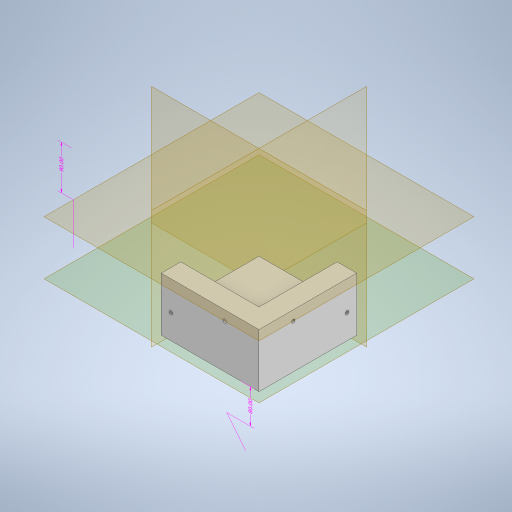
# Autodesk Inventor part: container_back_head_2
Saved by Autodesk Inventor 2023 (Build 270158000, 158)
## iProperties
Created: 2022-10-30
Part Number: container_back_head_2
Material: Genérico
Document SubType Name: Modeling
Designer: papel
Density: 1 g/cm^3
Appearance: Valor por defecto
Surface Area: 1564.19 cm^2
Author: papel
Autodesk Inventor part; units mm, degrees
ref_plane "YZ Plane" through (0, 0, 0) normal (1, 0, 0) x (0, 1, 0)
ref_plane "XZ Plane" through (0, 0, 0) normal (0, 1, 0) x (-1, 0, 0)
ref_plane "XY Plane" through (0, 0, 0) normal (0, 0, 1) x (1, 0, 0)
sketch "Boceto2" plane through (0, 0, 0) normal (0, 1, 0) x (-1, 0, 0)
  line L0 (7.5, 100) -> (-7.5, 100)
  line L1 (-7.5, 100) -> (-7.5, -100)
  line L2 (-7.5, -100) -> (7.5, -100)
  line L3 (7.5, -100) -> (7.5, 100)
  line L4 (7.5, 100) -> (-7.5, -100) construction
  line L5 (-7.5, 100) -> (7.5, -100) construction
  point P0 (0, 0)
  dimension "d7" = 15
  dimension "d8" = 200
  constraints: 12 end point, 2 midpoint, 2 parallel, 1 horizontal, 1 perpendicular
  measures "d7" distance of L2.end L1.end
  measures "d8" distance of L1.end L0.end
extrude "Extrusión1" add sketch "Boceto2" along normal blind 10
sketch "Boceto3" plane through (0, 10, 0) normal (0, 1, 0) x (1, 0, 0)
  line L0 (5, 60) -> (-5, 60)
  line L1 (-5, 60) -> (-5, 70)
  line L2 (-5, 70) -> (5, 70)
  line L3 (5, 70) -> (5, 60)
  line L4 (5, 60) -> (-5, 70) construction
  line L5 (7.5, 100) -> (-7.5, 100) projected
  line L6 (0, 64.5148) -> (0, 61.9205)
  circle A0 centre (3.25, 61.75) radius 1.75
  circle A1 centre (-3.25, 68.25) radius 1.75
  line L7 (-7.5, 100) -> (-7.5, -100) projected
  line L8 (-7.5, 0) -> (0, 0)
  line L9 (5, -70) -> (5, -60)
  line L10 (-5, -70) -> (5, -70)
  line L11 (5, -60) -> (-5, -60)
  line L12 (-5, -60) -> (-5, -70)
  line L13 (5, -60) -> (-5, -70) construction
  line L14 (0, -64.5148) -> (0, -61.9205)
  circle A2 centre (-3.25, -68.25) radius 1.75
  circle A3 centre (3.25, -61.75) radius 1.75
  point P0 (3.25, 68.25)
  point P1 (-5, 65)
  point P2 (-3.25, 61.75)
  point P3 (0, 100)
  point P4 (3.25, -68.25)
  point P5 (-3.25, -61.75)
  point P6 (-5, -65)
  dimension "d12" = 1.75
  dimension "d13" = 1.75
  dimension "d14" = 1.75
  dimension "d15" = 1.75
  dimension "d16" = 10
  dimension "d17" = 10
  dimension "d19" = 30
  dimension "d67" = 31.75
  constraints: 26 end point, 13 symmetric about line, 4 centre point, 3 midpoint, 2 horizontal, 2 parallel, 1 perpendicular, 1 vertical, 2 other
  measures "d12" distance from line of L2 point (3.25, 68.25)
  measures "d13" distance from line of L3 point (3.25, 68.25)
  measures "d14" distance from line of L1 point (-3.25, 61.75)
  measures "d15" distance from line of L0 point (-3.25, 61.75)
  measures "d16" distance between parallel lines of L0 L2
  measures "d17" distance between parallel lines of L3 L1
  measures "d19" distance from line of point (0, 100) L2
  measures "d67" distance from line of L5 A1.centre
hole "Agujero1" at (3.25, 10, -61.75) at (-3.25, 10, -68.25) at (-3.25, 10, 68.25) at (3.25, 10, 61.75) direction (0, -1, 0) diameter 3.5 end through all
sketch "Boceto4" plane through (0, 10, 0) normal (0, 1, 0) x (1, 0, 0)
  line L0 (-7.5, 100) -> (-7.5, -100) projected
  line L1 (-7.5, -100) -> (7.5, -100)
  line L2 (7.5, -100) -> (7.5, -80)
  line L3 (7.5, -80) -> (-7.5, -80)
  line L4 (-7.5, -80) -> (-7.5, -100)
  line L5 (-7.5, 0) -> (1.0116, 0)
  line L6 (-7.5, -100) -> (-7.5, 100)
  line L7 (-7.5, 100) -> (7.5, 100)
  line L8 (7.5, 100) -> (7.5, 80)
  line L9 (7.5, 80) -> (-7.5, 80)
  line L10 (-7.5, 80) -> (-7.5, 100)
  point P0 (0, 0)
  point P1 (-7.5, -80)
  point P2 (-7.5, 80)
  dimension "d27" = 15
  dimension "d28" = 20
  constraints: 20 end point, 5 symmetric about line, 2 horizontal, 2 parallel, 1 midpoint, 1 perpendicular
  measures "d27" distance of L3.end L2.end
  measures "d28" distance of L2.end L1.end
extrude "Extrusión2" add sketch "Boceto4" along normal blind 80
sketch "Boceto5" plane through (0, 90, 0) normal (0, 1, 0) x (1, 0, 0)
  line L0 (-7.5, -100) -> (7.5, -100) projected
  line L1 (-7.5, -100) -> (40.5, -100)
  line L2 (40.5, -100) -> (40.5, 100)
  line L3 (40.5, 100) -> (-7.5, 100)
  line L4 (-7.5, 100) -> (-7.5, -100)
  line L5 (40.5, -100) -> (-159.5, -100)
  line L6 (-159.5, -100) -> (-159.5, 100)
  line L7 (-159.5, 100) -> (40.5, 100)
  line L8 (40.5, 100) -> (40.5, -100)
  point P0 (0, 0)
  point P1 (-7.5, 100)
  dimension "d31" = 48
  dimension "d32" = 200
  dimension "d74" = 200
  constraints: 16 end point, 4 parallel, 2 horizontal, 2 perpendicular, 1 point on line
  measures "d31" distance of L3.end L2.end
  measures "d32" distance of L6.end L7.end
  measures "d74" distance between parallel lines of L7 L5
extrude "Extrusión3" add sketch "Boceto5" along normal blind 110
sketch "Boceto6" plane through (0, 200, 0) normal (0, 1, 0) x (1, 0, 0)
  line L0 (40.5, 100) -> (7.5, 100) projected
  line L1 (40.5, 100) -> (20.5, 100)
  line L2 (20.5, 100) -> (20.5, 80)
  line L3 (7.5, -100) -> (40.5, -100) projected
  line L4 (24, -100) -> (24, -80)
  line L5 (-159.5, 100) -> (-159.5, -100) projected
  line L6 (20.5, 80) -> (-159.5, 80)
  line L7 (-159.5, 80) -> (-159.5, -80)
  line L8 (-159.5, -80) -> (20.5, -80)
  line L9 (20.5, -80) -> (20.5, 80)
  line L10 (-159.5, -100) -> (40.5, -100) projected
  point P0 (7.5, 80)
  point P1 (-159.5, 80)
  dimension "d36" = 20
  dimension "d37" = 20
  dimension "d38" = 20
  dimension "d78" = 20
  constraints: 14 end point, 2 parallel, 2 perpendicular, 2 point on line, 1 horizontal, 1 midpoint, 1 vertical
  measures "d36" distance of L0.start L1.end
  measures "d37" distance of L1.end L2.end
  measures "d38" distance of L4.start L4.end
  measures "d78" distance between parallel lines of L10 L8
extrude "Extrusión4" cut sketch "Boceto6" against normal blind 90
sketch "Boceto7" plane through (-159.5, 90, -100) normal (-1, 0, 0) x (0, 0, 1)
  line L0 (0, 110) -> (20, 110) projected
  line L1 (20, 110) -> (10, 110)
  line L2 (10, 110) -> (10, 20)
  line L3 (10, 20) -> (20, 20)
  line L4 (20, 20) -> (20, 110)
  line L5 (180, 110) -> (180, 20) projected
  line L6 (180, 110) -> (190, 110)
  line L7 (190, 110) -> (190, 20)
  line L8 (190, 20) -> (180, 20)
  line L9 (180, 20) -> (180, 110)
  line L10 (200, 0) -> (200, 110) projected
  line L11 (0, 0) -> (0, 110) projected
  line L12 (0, 110) -> (10, 110)
  line L13 (10, 110) -> (10, 20)
  line L14 (10, 20) -> (0, 20)
  line L15 (0, 20) -> (0, 110)
  line L16 (200, 110) -> (0, 110) projected
  line L17 (200, 110) -> (190, 110)
  line L18 (190, 110) -> (190, 20)
  line L19 (190, 20) -> (200, 20)
  line L20 (200, 20) -> (200, 110)
  point P0 (100, -90)
  point P1 (200, 20)
  dimension "d42" = 10
  dimension "d63" = 10
  dimension "d65" = 10
  constraints: 32 end point, 8 parallel, 4 horizontal, 4 perpendicular, 1 point on line
  measures "d42" distance of L7.end L8.end
  measures "d63" distance between parallel lines of L10 L7
  measures "d65" distance between parallel lines of L11 L2
extrude "Extrusión5" cut sketch "Boceto7" against normal blind 30 contours L0 L2 L14 L11 | L16 L10 L19 L7
sketch "Boceto8" plane through (-7.5, 0, 100) normal (0, 0, 1) x (1, 0, 0)
  line L0 (-122, 200) -> (-122, 110) projected
  line L1 (-132, 175) -> (-142, 175)
  line L2 (-142, 175) -> (-142, 185)
  line L3 (-142, 185) -> (-132, 185)
  line L4 (-132, 185) -> (-132, 175)
  line L5 (-132, 175) -> (-142, 185) construction
  line L6 (-142, 175) -> (-132, 185) construction
  line L7 (-152, 200) -> (48, 200) projected
  line L8 (-113, 155) -> (-128, 155)
  line L9 (-152, 110) -> (-122, 110) projected
  line L10 (-132, 180) -> (-131.5898, 180)
  circle A0 centre (-140.25, 183.25) radius 1.75
  circle A1 centre (-133.75, 176.75) radius 1.75
  line L11 (-132, 125) -> (-132, 135)
  line L12 (-142, 125) -> (-132, 125)
  line L13 (-132, 135) -> (-142, 125) construction
  line L14 (-132, 135) -> (-142, 135)
  line L15 (-142, 135) -> (-132, 125) construction
  line L16 (-142, 135) -> (-142, 125)
  line L17 (-132, 130) -> (-131.5898, 130)
  circle A2 centre (-133.75, 133.25) radius 1.75
  circle A3 centre (-140.25, 126.75) radius 1.75
  line L18 (-152, 110) -> (-152, 200) projected
  point P0 (7.5, 0)
  point P1 (-113, 215)
  point P2 (-133.75, 183.25)
  point P3 (-142, 180)
  point P4 (-140.25, 176.75)
  point P5 (48, 200)
  point P6 (-133.75, 126.75)
  point P7 (-140.25, 133.25)
  point P8 (-143, 115)
  point P9 (-133.75, 126.75)
  point P10 (-140.25, 133.25)
  point P11 (-142, 130)
  dimension "d46" = 1.75
  dimension "d47" = 1.75
  dimension "d48" = 1.75
  dimension "d49" = 1.75
  dimension "d50" = 10
  dimension "d51" = 10
  dimension "d52" = 15
  dimension "d66" = 10
  dimension "d70" = 15
  constraints: 30 end point, 15 symmetric about line, 4 centre point, 3 horizontal, 2 midpoint, 2 parallel, 1 perpendicular, 5 other
  measures "d46" distance from line of L3 point (-133.75, 183.25)
  measures "d47" distance from line of L4 point (-133.75, 183.25)
  measures "d48" distance from line of L2 point (-140.25, 176.75)
  measures "d49" distance from line of L1 point (-140.25, 176.75)
  measures "d50" distance between parallel lines of L1 L3
  measures "d51" distance between parallel lines of L4 L2
  measures "d66" distance between parallel lines of L18 L2
hole "Agujero2" at (-147.75, 183.25, 100) at (-141.25, 176.75, 100) at (-147.75, 126.75, 100) at (-141.25, 133.25, 100) direction (0, 0, -1) diameter 3.5 end through all
ref_plane "Plano de trabajo1" through (-159.5, 90, 100) normal (0, -1, 0) x (1, 0, 0)
split "Dividir1" plane through (-159.5, 90, 100) removes the side toward (0, -1, 0)
ref_plane "Plano de trabajo2" through (-159.5, 200, 0) normal (0, 0, 1) x (1, 0, 0)
ref_plane "Plano de trabajo3" through (-59.5, 90, 100) normal (1, 0, 0) x (0, 0, -1)
sketch "Boceto9" plane through (-159.5, 90, 100) normal (0, 0, 1) x (1, 0, 0)
  line L0 (85.0357, 30) -> (115.0357, 30)
  circle A0 centre (110.0357, 25) radius 1.75
  line L1 (90.0357, 25) -> (110.0357, 25)
  line L2 (115.0357, 30) -> (115.0357, 20)
  circle A1 centre (90.0357, 25) radius 1.75
  line L3 (85.0357, 20) -> (115.0357, 30) construction
  line L4 (85.0357, 30) -> (115.0357, 20) construction
  line L5 (85.0357, 20) -> (85.0357, 30)
  line L6 (115.0357, 20) -> (85.0357, 20)
  line L7 (240, 0) -> (-40, 0) projected
  line L8 (200, 0) -> (200, 110) projected
  line L9 (200, 55) -> (88.2857, 55)
  line L10 (85.0357, 80) -> (115.0357, 80)
  circle A2 centre (110.0357, 85) radius 1.75
  line L11 (90.0357, 85) -> (110.0357, 85)
  line L12 (115.0357, 80) -> (115.0357, 90)
  circle A3 centre (90.0357, 85) radius 1.75
  line L13 (85.0357, 90) -> (115.0357, 80) construction
  line L14 (85.0357, 80) -> (115.0357, 90) construction
  line L15 (85.0357, 90) -> (85.0357, 80)
  line L16 (115.0357, 90) -> (85.0357, 90)
  line L17 (100.0357, 55) -> (185.099, 55) construction
  line L18 (160, 70) -> (160, 40)
  circle A4 centre (165, 45) radius 1.75
  line L19 (165, 65) -> (165, 45)
  line L20 (160, 40) -> (170, 40)
  circle A5 centre (165, 65) radius 1.75
  line L21 (170, 70) -> (160, 40) construction
  line L22 (160, 70) -> (170, 40) construction
  line L23 (170, 70) -> (160, 70)
  line L24 (170, 40) -> (170, 70)
  circle A6 centre (55, 65) radius 1.75
  line L25 (60, 70) -> (60, 40)
  line L26 (60, 70) -> (50, 40) construction
  line L27 (50, 70) -> (60, 70)
  line L28 (50, 40) -> (50, 70)
  line L29 (50, 70) -> (60, 40) construction
  circle A7 centre (55, 45) radius 1.75
  line L30 (55, 65) -> (55, 45)
  line L31 (60, 40) -> (50, 40)
  line L32 (30, 110) -> (30, 20) projected
  point P0 (159.5, -90)
  point P1 (100.0357, 34.7141)
  point P2 (85.0357, 36.6749)
  point P3 (100.0357, 34.7141)
  point P4 (115.0357, 25)
  point P5 (115.0357, 85)
  point P6 (189.1833, 40)
  point P7 (165, 70)
  point P8 (70.0357, 40)
  point P9 (55, 70)
  dimension "d83" = 10
  dimension "d84" = 30
  dimension "d85" = 5
  dimension "d86" = 5
  dimension "d87" = 5
  dimension "d88" = 5
  dimension "d89" = 20
  dimension "d91" = 30
  dimension "d92" = 5
  dimension "d93" = 5
  dimension "d94" = 3.5
  dimension "d95" = 5
  dimension "d96" = 5
  dimension "d97" = 5
  dimension "d98" = 5
  dimension "d99" = 5
  dimension "d100" = 20
  constraints: 54 end point, 8 centre point, 7 symmetric about line, 4 midpoint, 2 horizontal, 1 point on line, 11 other
  measures "d83" distance between parallel lines of L6 L0
  measures "d84" distance between parallel lines of L5 L2
  measures "d85" distance of point (115.036, 25) A0.centre
  measures "d86" distance from line of L0 A0.centre
  measures "d87" distance from line of L0 A1.centre
  measures "d88" distance from line of L5 A1.centre
  measures "d89" distance between parallel lines of L7 L6
  measures "d91" distance between parallel lines of L8 L24
  measures "d92" distance from line of L18 L19.start
  measures "d93" distance of point (165, 70) L19.start
  measures "d94" diameter of A4
  measures "d95" distance from line of L20 L19.end
  measures "d96" distance from line of L18 L19.end
  measures "d97" distance of point (55, 70) L30.start
  measures "d98" distance from line of L25 L30.end
  measures "d99" distance from line of L31 L30.end
  measures "d100" distance between parallel lines of L32 L28
ref_plane "Plano de trabajo4" through (0, 145, 0) normal (0, 1, 0) x (1, 0, 0)
hole "Agujero3" at (-104.5, 155, 100) at (-69.4643, 175, 100) at (-49.4643, 175, 100) at (-104.5, 135, 100) at (-69.4643, 115, 100) at (-49.4643, 115, 100) at (5.5, 135, 100) at (5.5, 155, 100) direction (0, 0, -1) diameter 3.5 end through all
sketch "Boceto10" plane through (40.5, 90, 100) normal (1, 0, 0) x (0, 0, -1)
  line L0 (85.0357, 30) -> (115.0357, 30)
  circle A0 centre (110.0357, 25) radius 1.75
  line L1 (90.0357, 25) -> (110.0357, 25)
  line L2 (115.0357, 30) -> (115.0357, 20)
  circle A1 centre (90.0357, 25) radius 1.75
  line L3 (85.0357, 20) -> (115.0357, 30) construction
  line L4 (85.0357, 30) -> (115.0357, 20) construction
  line L5 (85.0357, 20) -> (85.0357, 30)
  line L6 (115.0357, 20) -> (85.0357, 20)
  circle A2 centre (90.0357, 85) radius 1.75
  line L7 (85.0357, 80) -> (115.0357, 80)
  line L8 (85.0357, 80) -> (115.0357, 90) construction
  line L9 (85.0357, 90) -> (85.0357, 80)
  line L10 (115.0357, 90) -> (85.0357, 90)
  line L11 (85.0357, 90) -> (115.0357, 80) construction
  circle A3 centre (110.0357, 85) radius 1.75
  line L12 (90.0357, 85) -> (110.0357, 85)
  line L13 (115.0357, 80) -> (115.0357, 90)
  line L14 (160, 70) -> (160, 40)
  circle A4 centre (165, 45) radius 1.75
  line L15 (170, 40) -> (170, 70)
  line L16 (170, 70) -> (160, 40) construction
  line L17 (160, 40) -> (170, 40)
  line L18 (160, 70) -> (170, 40) construction
  circle A5 centre (165, 65) radius 1.75
  line L19 (165, 65) -> (165, 45)
  line L20 (170, 70) -> (160, 70)
  circle A6 centre (35, 65) radius 1.75
  line L21 (40, 70) -> (40, 40)
  line L22 (40, 40) -> (30, 40)
  circle A7 centre (35, 45) radius 1.75
  line L23 (35, 65) -> (35, 45)
  line L24 (40, 70) -> (30, 40) construction
  line L25 (30, 40) -> (30, 70)
  line L26 (30, 70) -> (40, 40) construction
  line L27 (30, 70) -> (40, 70)
  line L28 (0, 0) -> (0, 110) projected
  line L29 (200, 0) -> (200, 110) projected
  point P0 (100, -90)
  point P1 (100.0357, 34.7141)
  point P2 (100.0357, 34.7141)
  point P3 (85.0357, 36.6749)
  point P4 (115.0357, 25)
  point P5 (88.2857, 55)
  point P6 (115.0357, 85)
  point P7 (100.0357, 55)
  point P8 (189.1833, 40)
  point P9 (165, 70)
  point P10 (70.0357, 40)
  point P11 (35, 70)
  dimension "d108" = 10
  dimension "d109" = 30
  dimension "d110" = 5
  dimension "d111" = 5
  dimension "d112" = 5
  dimension "d113" = 5
  dimension "d114" = 5
  dimension "d115" = 5
  dimension "d116" = 3.5
  dimension "d117" = 5
  dimension "d118" = 5
  dimension "d119" = 5
  dimension "d120" = 5
  dimension "d121" = 5
  dimension "d122" = 30
  dimension "d123" = 30
  constraints: 50 end point, 8 centre point, 3 midpoint, 9 other
  measures "d108" distance between parallel lines of L6 L0
  measures "d109" distance between parallel lines of L5 L2
  measures "d110" distance of point (115.036, 25) A0.centre
  measures "d111" distance from line of L0 A0.centre
  measures "d112" distance from line of L0 A1.centre
  measures "d113" distance from line of L5 A1.centre
  measures "d114" distance from line of L14 L19.start
  measures "d115" distance of point (165, 70) L19.start
  measures "d116" diameter of A4
  measures "d117" distance from line of L17 L19.end
  measures "d118" distance from line of L14 L19.end
  measures "d119" distance of point (35, 70) L23.start
  measures "d120" distance from line of L21 L23.end
  measures "d121" distance from line of L22 L23.end
  measures "d122" distance between parallel lines of L28 L25
  measures "d123" distance between parallel lines of L29 L15
hole "Agujero4" at (40.5, 175, 9.9643) at (40.5, 175, -10.0357) at (40.5, 155, 65) at (40.5, 135, 65) at (40.5, 115, 9.9643) at (40.5, 115, -10.0357) at (40.5, 135, -65) at (40.5, 155, -65) direction (-1, 0, 0) diameter 3.5 end through all
split "Dividir2" plane through (-59.5, 90, 100) removes the side toward (-1, 0, 0)
split "Dividir3" plane through (0, 145, 0) removes the side toward (0, 1, 0)
split "Dividir4" plane through (-159.5, 200, 0) removes the side toward (0, 0, -1)
